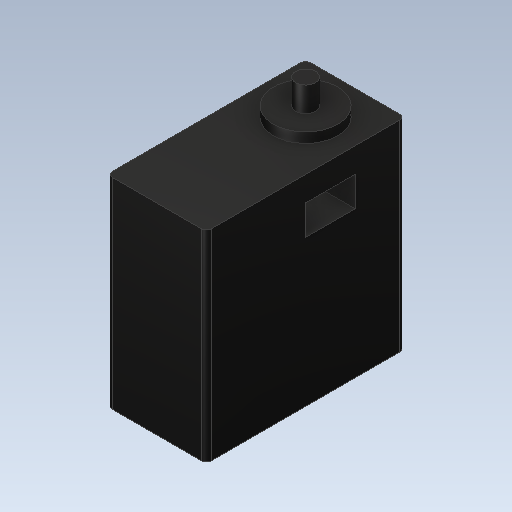
# Autodesk Inventor part: servo_FT_SC
Saved by Autodesk Inventor 2020.1 (Build 241239000, 239)
## iProperties
Created: 2017-12-03
Part Number: servo_FT_SC
Material: Generic
Document SubType Name: Modeling
Designer: Bardo91
Density: 1 g/cm^3
Appearance: Glossy - Black
Mass: 32.648 g
Surface Area: 65.7725 cm^2
Volume: 32.648 cm^3
Author: Bardo91
Autodesk Inventor part; units mm, degrees
ref_plane "YZ Plane" through (0, 0, 0) normal (1, 0, 0) x (0, 1, 0)
ref_plane "XZ Plane" through (0, 0, 0) normal (0, 1, 0) x (-1, 0, 0)
ref_plane "XY Plane" through (0, 0, 0) normal (0, 0, 1) x (1, 0, 0)
sketch "Sketch1" plane through (0, 0, 0) normal (0, 0, 1) x (1, 0, 0)
  line L0 (0, 0) -> (0, 40.5)
  line L1 (0, 40.5) -> (20, 40.5)
  line L2 (20, 40.5) -> (20, 0)
  line L3 (20, 0) -> (0, 0)
  dimension "d0" = 40.5
  dimension "d1" = 20
  constraints: 8 end point, 3 perpendicular, 1 vertical
  measures "d0" distance of L0.start L0.end
  measures "d1" distance of L0.end L1.end
extrude "Extrusion1" add sketch "Sketch1" along normal blind 40
sketch "Sketch2" plane through (0, 40.5, 0) normal (0, 1, 0) x (1, 0, 0)
  line L0 (20, 0) -> (0, 0) projected
  line L1 (10, 0) -> (10, -10)
  circle A0 centre (10, -10) radius 5
  dimension "d4" = 10
  dimension "d5" = 10
  constraints: 2 end point, 1 centre point, 1 coincident, 1 midpoint, 1 vertical
  measures "d4" distance of L1.start L1.end
  measures "d5" diameter of A0
extrude "Extrusion2" add sketch "Sketch2" along normal blind 1
sketch "Sketch3" plane through (10, 41.5, 10) normal (0, 1, 0) x (1, 0, 0)
  circle A0 centre (0, 0) radius 2
  point P0 (-10, 10)
  dimension "d8" = 4
  constraints: 1 centre point
  measures "d8" diameter of A0
extrude "Extrusion3" add sketch "Sketch3" along normal blind 6
fillet "Fillet1" radius 1 4 edges at (0, 20.25, 40) (20, 20.25, 40) (20, 20.25, 0) (0, 20.25, 0)
sketch "Sketch4" plane through (1, 0, 0) normal (0, -1, 0) x (1, 0, 0)
  line L0 (18, 0) -> (0, 0) projected
  line L1 (9, 0) -> (9, 10)
  circle A0 centre (9, 10) radius 5
  point P0 (-1, 0)
  dimension "d12" = 10
  dimension "d13" = 10
  constraints: 2 end point, 1 centre point, 1 coincident, 1 midpoint, 1 vertical
  measures "d12" distance of L1.start L1.end
  measures "d13" diameter of A0
extrude "Extrusion4" add sketch "Sketch4" along normal blind 1
sketch "Sketch5" plane through (10, -1, 10) normal (0, -1, 0) x (1, 0, 0)
  circle A0 centre (0, 0) radius 2
  point P0 (-10, -10)
  dimension "d16" = 4
  constraints: 1 centre point
  measures "d16" diameter of A0
extrude "Extrusion5" add sketch "Sketch5" along normal blind 4
sketch "Boceto6" plane through (0, 0, 1) normal (-1, 0, 0) x (0, 0, 1)
  line L0 (-1, 0) -> (-1, 40.5) projected
  line L1 (-1, 40.5) -> (-1, 35.5)
  line L2 (-1, 35.5) -> (9, 35.5)
  line L3 (9, 35.5) -> (9, 29.5)
  line L4 (9, 29.5) -> (19, 29.5)
  line L5 (19, 29.5) -> (19, 35.5)
  line L6 (19, 35.5) -> (9, 35.5)
  dimension "d19" = 5
  dimension "d20" = 10
  dimension "d21" = 6
  dimension "d22" = 10
  constraints: 12 end point, 5 perpendicular, 2 point on line
  measures "d19" distance of L0.end L1.end
  measures "d20" distance of L1.end L2.end
  measures "d21" distance of L2.end L3.end
  measures "d22" distance of L3.end L4.end
extrude "Extrusión6" cut sketch "Boceto6" against normal up to next
sketch "Boceto7" plane through (1, 0, 0) normal (0, -1, 0) x (1, 0, 0)
  line L0 (-1, 10) -> (19, 10) projected
  circle A0 centre (9, 10) radius 6.5
  circle A1 centre (9, 10) radius 2
  point P0 (-1, 0)
  dimension "d25" = 13
  constraints: 2 centre point, 1 coincident, 1 midpoint
  measures "d25" diameter of A0
extrude "Extrusión8" add sketch "Boceto7" along normal blind 2 contours A1 L0 A0 | L0 A0 A1
sketch "Boceto8" plane through (1, 40.5, 0) normal (0, 1, 0) x (1, 0, 0)
  circle A0 centre (9, -10) radius 2 projected
  circle A1 centre (9, -10) radius 6.5
  circle A2 centre (9, -10) radius 6.5 projected
  circle A3 centre (9, -10) radius 2
  point P0 (-1, 0)
  dimension "d30" = 13
  constraints: 2 centre point, 2 coincident, 1 concentric
  measures "d30" diameter of A1
extrude "Extrusión9" add sketch "Boceto8" along normal blind 2
body "Solid1"
